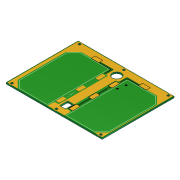
# Autodesk Inventor part: FOX-ME-119-05
Saved by Autodesk Inventor 2014 (Build 180170000, 170)
## iProperties
Created: 2011-02-15
Material: FR4
Document SubType Name: Modeling
Designer: Robert Davis
Mass: 17.526 g
Surface Area: 165.715 cm^2
Volume: 12.7 cm^3
Density: 2.04 g/cm^3
Description: PCB
Part Number: FOX-ME-119-05
Appearance: Olive Green
Author: Robert Davis
Autodesk Inventor part; units mm, degrees
ref_plane "YZ Plane" through (0, 0, 0) normal (1, 0, 0) x (0, 1, 0)
ref_plane "XZ Plane" through (0, 0, 0) normal (0, 1, 0) x (-1, 0, 0)
ref_plane "XY Plane" through (0, 0, 0) normal (0, 0, 1) x (1, 0, 0)
sketch "Sketch1" plane through (0, 0, 0) normal (0, 0, 1) x (1, 0, 0)
  line L0 (-54, -40.5) -> (54, -40.5)
  line L1 (54, -40.5) -> (54, 40.5)
  line L2 (54, 40.5) -> (-54, 40.5)
  line L3 (-54, 40.5) -> (-54, -40.5)
  point P0 (0, 0)
  dimension "d0" = 108
  dimension "d1" = 81
  dimension "d2" = 40.5
  dimension "d3" = 54
  constraints: 8 end point, 2 horizontal, 2 vertical
  measures "d0" distance of L1.end L2.end
  measures "d1" distance of L0.end L1.end
  measures "d2" distance from line of point (0, 0) L2
  measures "d3" distance from line of L1 point (0, 0)
extrude "Extrusion1" add sketch "Sketch1" along normal blind 1.5875
hole "Hole2" at (50, -38, 1.5875) direction (0, 0, -1) diameter 2.6924 end through all
mirror "Mirror1" about plane through (0, 0, 0) normal (0, 1, 0) of "Hole2"
hole "Hole_audio" at (1.4, 28.5, 1.5875) direction (0, 0, -1) diameter 9.525 end through all
hole "Hole_mini_usb" [suppressed]
mirror "Mirror2" about plane through (0, 0, 0) normal (1, 0, 0) of "Hole2", "Mirror1"
hole "Hole5" at (0, -38, 1.5875) direction (0, 0, -1) diameter 2.6924 end through all
mirror "Mirror3" about plane through (0, 0, 0) normal (0, 1, 0) of "Hole5"
hole "Hole6" [suppressed]
mirror "Mirror4" [suppressed]
sketch "Sketch2" plane through (0, 0, 0) normal (0, 0, -1) x (-1, 0, 0)
  line L0 (-0.4125, -24.055) -> (-3.5875, -24.055)
  line L1 (-5.175, -25.6425) -> (-5.175, -31.3575)
  line L2 (-3.5875, -32.945) -> (-0.4125, -32.945)
  line L3 (1.175, -31.3575) -> (1.175, -25.6425)
  line L4 (-2, -22.5163) -> (-2, -34.6324)
  line L5 (-9.4902, -28.5) -> (-22.3716, -28.5)
  arc A0 (-0.4125, -32.945) -> (1.175, -31.3575) centre (-0.4125, -31.3575) ccw
  arc A1 (-5.175, -31.3575) -> (-3.5875, -32.945) centre (-3.5875, -31.3575) ccw
  arc A2 (-3.5875, -24.055) -> (-5.175, -25.6425) centre (-3.5875, -25.6425) ccw
  arc A3 (1.175, -25.6425) -> (-0.4125, -24.055) centre (-0.4125, -25.6425) ccw
  line L6 (54, -40.5) -> (-54, -40.5) projected
  point P0 (0, 0)
  point P1 (1.175, -24.055)
  point P2 (-5.175, -32.945)
  point P3 (1.175, -32.945)
  point P4 (-2, -28.5)
  dimension "d80" = 6.35
  dimension "d81" = 8.89
  dimension "d82" = 1.5875
  dimension "d85" = 12
  dimension "d87" = 2
  constraints: 12 end point, 8 point on circle, 8 point on line, 8 tangent, 4 centre point, 3 equal radius, 1 horizontal, 1 vertical, 2 other
  measures "d80" distance of point (-5.175, -32.945) point (1.175, -32.945)
  measures "d81" distance of point (1.175, -32.945) point (1.175, -24.055)
  measures "d82" radius of A0
  measures "d85" distance from line of L6 point (-2, -28.5)
  measures "d87" horizontal distance of point (0, 0) point (-2, -28.5)
extrude "cutout_mini_usb" cut sketch "Sketch2" against normal through all
sketch "Sketch4" plane through (0, 0, 1.5875) normal (0, 0, 1) x (1, 0, 0)
  line L0 (-54, -40.5) -> (-54, 40.5) projected
  line L1 (54, -40.5) -> (-54, -40.5) projected
  line L2 (54, 40.5) -> (54, -40.5) projected
  line L3 (-54, 40.5) -> (54, 40.5) projected
  line L4 (-53.878, -40.6622) -> (-54, 40.5) construction
  line L5 (-54, 40.5) -> (53.878, 40.6622) construction
  line L6 (53.878, 40.6622) -> (54, -40.5) construction
  line L7 (54, -40.5) -> (-53.878, -40.6622) construction
  point P0 (0, 0)
  constraints: 4 point on line, 2 other
decal "Decal1"
sketch "Sketch5" plane through (0, 0, 0) normal (0, 0, -1) x (-1, 0, 0)
  line L0 (54, -40.5) -> (-54, -40.5) projected
  line L1 (54, 40.5) -> (54, -40.5) projected
  line L2 (-54, 40.5) -> (54, 40.5) projected
  line L3 (-54, -40.5) -> (-54, 40.5) projected
  line L4 (53.9396, 40.5804) -> (54, -40.5) construction
  line L5 (54, -40.5) -> (-53.9396, -40.5804) construction
  line L6 (-53.9396, -40.5804) -> (-54, 40.5) construction
  line L7 (-54, 40.5) -> (53.9396, 40.5804) construction
  point P0 (0, 0)
  constraints: 4 point on line, 2 other
decal "Decal2"
body "Solid1"
